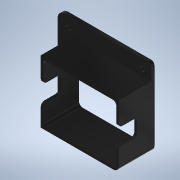
# Autodesk Inventor part: SP49V1 Protector Pasador
Saved by Autodesk Inventor 2021.2 (Build 252289000, 289)
## iProperties
Created: 2026-09-07
Part Number: SP49V1 Protector Pasador
Material: ABS Plastic
Document SubType Name: Modeling
Designer: nelso
Density: 1.06 g/cm^3
Appearance: Smooth - Black
Author: nelso
Autodesk Inventor part; units mm, degrees
ref_plane "YZ Plane" through (0, 0, 0) normal (1, 0, 0) x (0, 1, 0)
ref_plane "XZ Plane" through (0, 0, 0) normal (0, 1, 0) x (-1, 0, 0)
ref_plane "XY Plane" through (0, 0, 0) normal (0, 0, 1) x (1, 0, 0)
sketch "Sketch1" plane through (0, 0, 0) normal (0, 1, 0) x (-1, 0, 0)
  line L0 (32.35, 26) -> (-32.35, 26)
  line L1 (-32.35, 26) -> (-32.35, -26)
  line L2 (-32.35, -26) -> (32.35, -26)
  line L3 (32.35, -26) -> (32.35, 26)
  line L4 (32.35, 26) -> (-32.35, -26) construction
  line L5 (-32.35, 26) -> (32.35, -26) construction
  point P0 (0, 0)
  dimension "d0" = 64.7
  dimension "d1" = 52
  constraints: 12 end point, 2 midpoint, 2 parallel, 1 horizontal, 1 perpendicular
  measures "d0" distance of L2.end L1.end
  measures "d1" distance of L1.end L0.end
extrude "Extrusion1" add sketch "Sketch1" along normal mid plane 30
shell "Shell1" thickness 2 removed faces 2 at (10.7833, 15, 8.6667) at (10.7833, -15, 8.6667)
sketch "Sketch3" plane through (32.35, -15, 26) normal (1, 0, 0) x (0, 0, -1)
  line L0 (0, 30) -> (0, 0) projected
  line L1 (0, 0) -> (19.9, 0)
  line L2 (2, 0) -> (50, 0) projected
  line L3 (19.9, 0) -> (33.9, 0)
  line L4 (33.9, 0) -> (33.9, 15)
  line L5 (33.9, 15) -> (19.9, 15)
  line L6 (19.9, 15) -> (19.9, 0)
  point P0 (26, 15)
  point P1 (0, 27)
  point P2 (33.9, 0)
  dimension "d12" = 19.9
  dimension "d13" = 14
  dimension "d14" = 15
  constraints: 10 end point, 2 parallel, 1 horizontal, 1 perpendicular, 1 point on line
  measures "d12" distance of L0.end L1.end
  measures "d13" distance of L5.end L4.end
  measures "d14" distance of L4.end L3.end
extrude "Extrusion3" cut sketch "Sketch3" against normal through all
sketch "Sketch4" plane through (0, 15, 0) normal (0, 1, 0) x (1, 0, 0)
  line L0 (32.35, -26) -> (32.35, 26) projected
  line L1 (30.35, -24) -> (-30.35, -24) projected
  line L2 (32.35, 26) -> (-30.35, 26)
  line L3 (-30.35, 26) -> (-30.35, -24)
  line L4 (-30.35, -24) -> (32.35, -24)
  line L5 (32.35, -24) -> (32.35, 26)
  line L6 (32.35, 26) -> (-32.35, 26) projected
  line L7 (32.35, 26) -> (-45.35, 26)
  line L8 (-45.35, 26) -> (-45.35, -39)
  line L9 (-45.35, -39) -> (32.35, -39)
  line L10 (32.35, -39) -> (32.35, 26)
  point P0 (0, 0)
  dimension "d17" = 77.7
  dimension "d18" = 65
  constraints: 16 end point, 4 parallel, 2 horizontal, 2 perpendicular
  measures "d17" distance of L9.end L8.end
  measures "d18" distance of L8.end L7.end
extrude "Extrusion4" add sketch "Sketch4" against normal blind 3 contours L10 L9 L8 L7 L6 L3 L1 L4 L0
fillet "Fillet1" radius 3 14 edges at (-30.35, 0, 24) (-30.35, 0, -24) (-31.35, 0, -7.9) (-31.35, 0, 6.1) (31.35, 0, -7.9) (31.35, 0, 6.1) (30.35, 0, -24) (30.35, 0, 24) (32.35, 13.5, 39) (-45.35, 13.5, -26) (-31.35, -15, -7.9) (-31.35, -15, 6.1) (31.35, -15, 6.1) (31.35, -15, -7.9)
fillet "Fillet1" radius 6 1 edges at (-45.35, 13.5, 39)
fillet "Fillet1" radius 4.5 1 edges at (32.35, 0, -26)
sketch "Sketch5" plane through (0, 15, 0) normal (0, 1, 0) x (1, 0, 0)
  line L0 (-30.35, -21) -> (-30.35, 21) projected
  line L1 (-45.35, 26) -> (-30.35, 26)
  line L2 (-30.35, 26) -> (-30.35, 11)
  line L3 (-30.35, 11) -> (-45.35, 11)
  line L4 (-45.35, 11) -> (-45.35, 26)
  arc A0 (-30.35, -21) -> (-27.35, -24) centre (-27.35, -21) ccw projected
  line L5 (-45.35, -39) -> (-27.35, -39)
  line L6 (-27.35, -39) -> (-27.35, -21)
  line L7 (-27.35, -21) -> (-45.35, -21)
  line L8 (-45.35, -21) -> (-45.35, -39)
  line L9 (27.35, -24) -> (-27.35, -24) projected
  line L10 (32.35, -39) -> (17.35, -39)
  line L11 (17.35, -39) -> (17.35, -24)
  line L12 (17.35, -24) -> (32.35, -24)
  line L13 (32.35, -24) -> (32.35, -39)
  point P0 (0, 0)
  point P1 (-37.85, 18.5)
  point P2 (-36.35, -30)
  point P3 (24.85, -31.5)
  dimension "d23" = 15
  dimension "d24" = 15
  constraints: 24 end point, 6 parallel, 4 point on line, 3 horizontal, 3 perpendicular
  measures "d23" distance of L1.end L2.end
  measures "d24" distance of L11.end L12.end
hole "Hole1" at (-37.85, 15, -18.5) at (-36.35, 15, 30) at (24.85, 15, 31.5) direction (0, -1, 0) diameter 3.6 depth 8 tip angle 118 clearance for "Countersunk Flat Head Screw ISO 2009/7046" size "M3" standard "ISO"
chamfer "Chamfer1" distance 0.3 angle 45 19 edges at (-7.25, 15, -26) (-44.4713, 15, -25.1213) (-45.35, 15, 5) (-43.5926, 15, 37.2426) (-5, 15, 39) (31.4713, 15, 38.1213) (32.35, 15, 7.25) (31.032, 15, -24.682) (-29.4713, 15, -23.1213) (-30.35, 15, 0) (-29.4713, 15, 23.1213) (0, 15, 24) (29.4713, 15, 23.1213) (30.35, 15, 0) (29.4713, 15, -23.1213) (0, 15, -24) (-37.85, 15, -20.3) (-36.35, 15, 28.2) (24.85, 15, 29.7)
body "Solid1"
